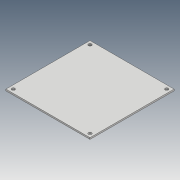
# Autodesk Inventor part: 제어회로
Saved by Autodesk Inventor 2018 (Build 220112000, 112)
## iProperties
Created: 2018-10-26
Part Number: 제어회로
Material: 일반
Document SubType Name: Modeling
Designer: dhksr
Density: 1 g/cm^3
Appearance: 기본값
Author: dhksr
Autodesk Inventor part; units mm, degrees
ref_plane "YZ Plane" through (0, 0, 0) normal (1, 0, 0) x (0, 1, 0)
ref_plane "XZ Plane" through (0, 0, 0) normal (0, 1, 0) x (-1, 0, 0)
ref_plane "XY Plane" through (0, 0, 0) normal (0, 0, 1) x (1, 0, 0)
sketch "스케치1" plane through (0, 0, 0) normal (0, 0, 1) x (1, 0, 0)
  line L0 (40, 40) -> (-40, 40)
  line L1 (-40, 40) -> (-40, -40)
  line L2 (-40, -40) -> (40, -40)
  line L3 (40, -40) -> (40, 40)
  line L4 (40, 40) -> (-40, -40) construction
  line L5 (-40, 40) -> (40, -40) construction
  line L6 (36.5, -36.5) -> (-36.5, -36.5) construction
  line L7 (-36.5, -36.5) -> (-36.5, 36.5) construction
  line L8 (-36.5, 36.5) -> (36.5, 36.5) construction
  line L9 (36.5, 36.5) -> (36.5, -36.5) construction
  line L10 (36.5, -36.5) -> (-36.5, 36.5) construction
  line L11 (-36.5, -36.5) -> (36.5, 36.5) construction
  circle A0 centre (-36.5, 36.5) radius 1.5
  circle A1 centre (-36.5, -36.5) radius 1.5
  circle A2 centre (36.5, -36.5) radius 1.5
  circle A3 centre (36.5, 36.5) radius 1.5
  point P0 (0, 0)
  dimension "d0" = 80
  dimension "d1" = 80
  dimension "d2" = 73
  dimension "d3" = 73
  dimension "d4" = 3
  dimension "d5" = 3
  dimension "d6" = 3
  dimension "d7" = 3
  constraints: 24 end point, 4 centre point, 4 coincident, 4 midpoint, 4 parallel, 2 horizontal, 2 perpendicular
  measures "d0" distance of L2.end L1.end
  measures "d1" distance of L1.end L0.end
  measures "d2" distance of L7.end L8.end
  measures "d3" distance of L6.end L7.end
  measures "d4" diameter of A0
  measures "d5" diameter of A1
  measures "d6" diameter of A2
  measures "d7" diameter of A3
extrude "돌출1" add sketch "스케치1" along normal blind 1.5
